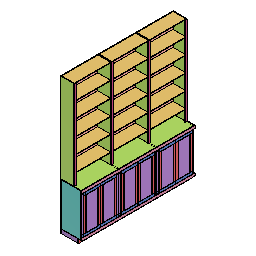
MS_BookShelves (Autodesk Fusion 360 design; units mm, degrees)
description: 68.5"x10"x0.5"
description: 10"x28"x0.5"
description: 87"x16"x0.5"
description: 29"x3"x0.5"
description: 13"x3"x0.5"
description: 6"x3"x1.5"
description: 29"x14"0.5"
description: 32.75"x13"x0.5"
description: 32.75"x29"x0.5"
description: 26.75"x3"x0.5"
description: 68.5"x29"x0.5"
description: 12.875"x2"x0.5"
description: 25.75"x2"0.5"
description: 26"x9.125"x0.25"
description: 87.5"x1.75"x0.5"
description: 16.5"x1.75"x0.5"
description: 68.5"x1.5"x0.5"
Autodesk Fusion 360 part; units mm, degrees
sketch "Sketch2" plane through (0, 0, 0) normal (0, 0, 1) x (1, 0, 0)
  line L0 (0, 0) -> (254, 0)
  line L1 (254, 0) -> (254, 2263.775)
  line L2 (254, 2263.775) -> (0, 2263.775)
  line L3 (0, 2263.775) -> (0, 0)
  line L4 (0, 0) -> (406.4, 0)
  line L5 (406.4, 0) -> (406.4, 2263.775)
  line L6 (406.4, 2263.775) -> (0, 2263.775)
  line L7 (0, 2263.775) -> (0, 0)
  line L8 (406.4, 0) -> (1338.2625, 0)
  line L9 (1338.2625, 0) -> (1338.2625, 406.4)
  line L10 (1338.2625, 406.4) -> (406.4, 406.4)
  line L11 (406.4, 406.4) -> (406.4, 0)
  dimension "d42" = 254
  dimension "d43" = 2263.775
  dimension "d45" = 406.4
  dimension "d46" = 2263.775
  dimension "d48" = 931.8625
  dimension "d49" = 406.4
  constraint horizontal L0
  constraint vertical L1
  constraint horizontal L2
  constraint vertical L3
  constraint coincident L0.start L3.end
  constraint horizontal L4
  constraint vertical L5
  constraint horizontal L6
  constraint vertical L7
  constraint horizontal L8
  constraint vertical L9
  constraint horizontal L10
  constraint vertical L11
  measures "d42" distance of L0.start L0.end
  measures "d43" distance of L0.start L2.end
  measures "d45" distance of L0.start L4.end
  measures "d46" distance of L0.start L2.end
  measures "d48" distance of L4.end L8.end
  measures "d49" distance of L4.end L10.end
sketch "Sketch1" plane through (0, 0, 0) normal (0, 0, 1) x (1, 0, 0) in component "Room"
  line L0 (0, 0) -> (3648.075, 0)
  line L1 (2259.0125, 0) -> (1363.6625, 0) construction
  line L2 (1363.6625, 0) -> (1363.6625, 46.449) construction
  line L3 (1363.6625, 46.449) -> (2259.0125, 46.449) construction
  line L4 (2259.0125, 46.449) -> (2259.0125, 0) construction
  line L5 (0, 0) -> (0, 3178.175)
  line L6 (0, 3178.175) -> (922.3375, 3178.175)
  line L7 (922.3375, 3178.175) -> (2225.675, 3178.175)
  line L8 (2225.675, 3178.175) -> (3114.675, 3178.175)
  line L9 (3114.675, 3178.175) -> (3630.6125, 3178.175)
  line L10 (0, 2403.475) -> (58.5758, 2403.475) construction
  line L11 (58.5758, 2403.475) -> (58.5758, 2317.75) construction
  line L12 (58.5758, 2317.75) -> (0, 2317.75) construction
  line L13 (0, 2317.75) -> (0, 2403.475) construction
  line L14 (140.5097, 3178.175) -> (140.5097, 2420.9375) construction
  point P0 (1363.6625, 0)
  point P1 (2259.0125, 0)
  point P2 (0, 2403.475)
  point P3 (0, 2317.75)
  dimension "d18" = 3648.075
  dimension "d19" = 895.35
  dimension "d20" = 1363.6625
  dimension "d21" = 1389.0625
  dimension "d22" = 3178.175
  dimension "d23" = 922.3375
  dimension "d24" = 1303.3375
  dimension "d25" = 889
  dimension "d26" = 515.9375
  dimension "d27" = 3630.6125
  dimension "d34" = 774.7
  dimension "d35" = 85.725
  dimension "d36" = 757.2375
  dimension "d37" = 90
  constraint coincident L0.start L5.start
  constraint horizontal L0
  constraint coincident L0 P0
  constraint coincident L0 P1
  constraint horizontal L1
  constraint vertical L2
  constraint horizontal L3
  constraint vertical L4
  constraint coincident P1 L1.start
  constraint perpendicular L0 L5
  constraint perpendicular L5 L6
  constraint parallel L6 L7
  constraint parallel L7 L8
  constraint parallel L8 L9
  constraint coincident L5 P2
  constraint coincident L5 P3
  constraint horizontal L10
  constraint vertical L11
  constraint horizontal L12
  constraint vertical L13
  constraint coincident P2 L10.start
  constraint coincident L6 L14.start
  constraint perpendicular L6 L14
  measures "d18" distance of L0.start L0.end
  measures "d19" distance of P0 P1
  measures "d20" distance of L0.start L1.end
  measures "d21" distance of L0.end P1
  measures "d22" distance of L0.start L5.end
  measures "d23" distance of L5.end L6.end
  measures "d24" distance of L6.end L7.end
  measures "d25" distance of L7.end L8.end
  measures "d26" distance of L8.end L9.end
  measures "d27" distance of L5.end L9.end
  measures "d34" distance of L5.end P2
  measures "d35" distance of P2 P3
  measures "d36" distance of L14.start L14.end
  measures "d37" angle of L6 L14
sketch "Sketch1 (2)" plane through (0, 0, 0) normal (1, 0, 0) x (0, 1, 0) in component "Shelves"
  line L0 (12.7, 2667) -> (723.9, 2667)
  line L1 (723.9, 2667) -> (723.9, 2654.3)
  line L2 (723.9, 2654.3) -> (12.7, 2654.3)
  line L3 (12.7, 2654.3) -> (12.7, 2667)
  point P0 (0, 914.4)
  point P1 (0, 927.1)
  point P2 (0, 76.2)
  point P3 (0, 2667)
  point P4 (12.7, 2667)
  dimension "d51" = 12.7
  dimension "d54" = 76.2
  dimension "d55" = 838.2
  dimension "d56" = 1739.9
  dimension "d76" = 12.7
  dimension "d77" = 711.2
  dimension "d78" = 12.7
  constraint horizontal L0
  constraint vertical L1
  constraint horizontal L2
  constraint vertical L3
  constraint coincident P4 L0.start
  measures "d51" distance of P0 P1
  measures "d54" distance of P2 origin
  measures "d55" distance of P0 P2
  measures "d56" distance of P1 P3
  measures "d76" distance of P3 P4
  measures "d77" distance of P4 L0.end
  measures "d78" distance of P4 L2.end
ref_plane "WorkPlane1" through (0, 0, 2743.2) normal (0, 0, 1) x (1, 0, 0) in component "Room"
sketch "Sketch1 (1)" plane through (0, 0, 2743.2) normal (0, 0, 1) x (1, 0, 0) in component "Room"
  line L0 (0, 0) -> (3648.075, 0) construction
  line L1 (3648.075, 0) -> (3648.075, 3178.175) construction
  line L2 (3648.075, 3178.175) -> (0, 3178.175) construction
  line L3 (0, 3178.175) -> (0, 0) construction
  dimension "d58" = 3648.075
  dimension "d59" = 3178.175
  constraint horizontal L0
  constraint vertical L1
  constraint horizontal L2
  constraint vertical L3
  constraint coincident L0.start L3.end
  measures "d58" distance of L0.start L0.end
  measures "d59" distance of L0.start L2.end
sketch "Sketch1 (3)" plane through (0, 0, 0) normal (0, 1, 0) x (1, 0, 0) in component "Shelf Sides"
  line L0 (0, -927.1) -> (260.35, -927.1)
  line L1 (260.35, -927.1) -> (260.35, -2667)
  line L2 (260.35, -2667) -> (0, -2667)
  line L3 (0, -2667) -> (0, -927.1)
  point P0 (0, -927.1)
  dimension "d60" = 260.35
  dimension "d61" = 1739.9
  constraint horizontal L0
  constraint vertical L1
  constraint horizontal L2
  constraint vertical L3
  constraint coincident P0 L0.start
  measures "d60" distance of P0 L0.end
  measures "d61" distance of P0 L2.end
extrude "Extrude1" add sketch "Sketch1 (3)" along normal blind 12.7 makes body 1 in component "Shelf Sides"
pattern_linear "00000000-0000-0000-0000-000000000000" [suppressed] in component "Shelves"
extrude "Extrude1'" add sketch "Sketch1 (2)" along normal blind 254 separate body makes body 2 in component "Shelves (1)"
sketch "Sketch1 (4)" plane through (6.35, 0, 0) normal (-1, 0, 0) x (0, -1, 0) in component "Shelf Back"
  line L0 (0, 927.1) -> (0, 2667)
  line L1 (0, 2667) -> (-12.7, 2667)
  line L2 (-12.7, 2667) -> (-12.7, 927.1)
  line L3 (-12.7, 927.1) -> (0, 927.1)
  line L4 (0, 927.1) -> (-736.6, 927.1)
  line L5 (-736.6, 927.1) -> (-736.6, 2667)
  line L6 (-736.6, 2667) -> (0, 2667)
  line L7 (0, 2667) -> (0, 927.1)
  line L8 (-723.9, 939.8) -> (-723.9, 2654.3)
  line L9 (-723.9, 2654.3) -> (-12.7, 2654.3)
  line L10 (-12.7, 2654.3) -> (-12.7, 939.8)
  line L11 (-12.7, 939.8) -> (-723.9, 939.8)
  line L12 (-723.9, 939.8) -> (-723.9, 927.1)
  line L13 (-12.7, 939.8) -> (-12.7, 927.1)
  line L14 (-723.9, 927.1) -> (-723.9, 2667)
  line L15 (-723.9, 2667) -> (-736.6, 2667)
  line L16 (-736.6, 2667) -> (-736.6, 927.1)
  line L17 (-736.6, 927.1) -> (-723.9, 927.1)
  line L18 (-723.9, 2654.3) -> (-12.7, 2654.3)
  line L19 (-12.7, 2654.3) -> (-12.7, 2667)
  line L20 (-12.7, 2667) -> (-723.9, 2667)
  line L21 (-723.9, 2667) -> (-723.9, 2654.3)
  line L22 (-723.9, 2654.3) -> (-12.7, 2654.3)
  line L23 (-12.7, 2654.3) -> (-12.7, 2667)
  line L24 (-12.7, 2667) -> (-723.9, 2667)
  line L25 (-723.9, 2667) -> (-723.9, 2654.3)
  dimension "d215" = 736.6
  dimension "d216" = 1739.9
  dimension "d217" = 12.7
  dimension "d220" = 12.7
  dimension "d221" = 12.7
  constraint horizontal L4
  constraint vertical L5
  constraint horizontal L6
  constraint vertical L7
  constraint coincident L0.start L3.end
  constraint perpendicular L11 L12
  constraint perpendicular L11 L13
  measures "d215" distance of L0.start L4.end
  measures "d216" distance of L0.start L0.end
  measures "d220" distance of L8.start L12.end
  measures "d221" distance of L10.end L2.end
extrude "Extrude1''" add sketch "Sketch1 (4)" against normal blind 6.35 separate body contours L2 L4 L11 L12 L13 L14 | L2 L8 L9 L10 L11 L14 L18 L22 makes body 3 in component "Shelf Back"
extrude "Extrude3" add sketch "Sketch1 (4)" along normal blind 6.35 separate body makes body 4 in component "Shelf Back"
pattern_linear "00000000-0000-0000-0000-000000000000'" [suppressed] in component "Shelves"
pattern_linear "00000000-0000-0000-0000-000000000000''" [suppressed] in component "Shelves"
pattern_linear "00000000-0000-0000-0000-000000000000'''" [suppressed] in component "Shelves"
pattern_linear "00000000-0000-0000-0000-000000000000''''" [suppressed] in component "Shelves"
sketch "Sketch1 (5)" plane through (0, 0, 0) normal (1, 0, 0) x (0, 1, 0) in component "Cabinet Tbl Top"
  line L0 (0, 914.4) -> (2209.8, 914.4)
  line L1 (2209.8, 914.4) -> (2209.8, 927.1)
  line L2 (2209.8, 927.1) -> (0, 927.1)
  line L3 (0, 927.1) -> (0, 914.4)
  point P0 (0, 76.2)
  point P1 (0, 914.4)
  point P2 (0, 76.2)
  dimension "d101" = 76.2
  dimension "d102" = 838.2
  dimension "d103" = 2209.8
  dimension "d104" = 12.7
  constraint vertical P0 L0.start
  constraint horizontal L0
  constraint vertical L1
  constraint horizontal L2
  constraint vertical L3
  constraint coincident P1 L0.start
  measures "d101" distance of P2 origin
  measures "d102" distance of P1 P0
  measures "d103" distance of P1 L0.end
  measures "d104" distance of P1 L2.end
extrude "Extrude1'''" add sketch "Sketch1 (5)" along normal blind 406.4 separate body makes body 5 in component "Cabinet Tbl Top"
sketch "Sketch1 (6)" plane through (0, 0, 0) normal (0, 0, 1) x (1, 0, 0) in component "Toe Guard"
  line L0 (0, 0) -> (12.7, 0)
  line L1 (12.7, 0) -> (12.7, 736.6)
  line L2 (12.7, 736.6) -> (0, 736.6)
  line L3 (0, 736.6) -> (0, 0)
  line L4 (0, 0) -> (406.4, 0)
  line L5 (342.9, 0) -> (355.6, 0)
  line L6 (355.6, 0) -> (355.6, 736.6)
  line L7 (355.6, 736.6) -> (342.9, 736.6)
  line L8 (342.9, 736.6) -> (342.9, 0)
  line L9 (12.7, 736.6) -> (342.9, 736.6)
  line L10 (342.9, 736.6) -> (342.9, 723.9)
  line L11 (342.9, 723.9) -> (12.7, 723.9)
  line L12 (12.7, 723.9) -> (12.7, 736.6)
  line L13 (12.7, 0) -> (342.9, 0)
  line L14 (342.9, 0) -> (342.9, 12.7)
  line L15 (342.9, 12.7) -> (12.7, 12.7)
  line L16 (12.7, 12.7) -> (12.7, 0)
  line L17 (120.4631, 12.7) -> (12.7, 120.4631)
  line L18 (75.5618, 3.7197) -> (3.7197, 75.5618)
  line L19 (177.8, 368.3, 0) -> (177.8, 368.3, 108.5578) construction
  point P0 (342.9, 0)
  point P1 (12.7, 12.7)
  point P2 (120.4631, 12.7)
  point P3 (12.7, 120.4631)
  point P4 (342.9, 368.3)
  point P5 (177.8, 12.7)
  point P6 (177.8, 368.3)
  dimension "d107" = 12.7
  dimension "d108" = 736.6
  dimension "d114" = 330.2
  dimension "d115" = 12.7
  dimension "d116" = 736.6
  dimension "d117" = 330.2
  dimension "d118" = 12.7
  dimension "d119" = 330.2
  dimension "d120" = 12.7
  dimension "d138" = 45
  dimension "d139" = 152.4
  constraint horizontal L0
  constraint vertical L1
  constraint horizontal L2
  constraint vertical L3
  constraint coincident L0.start L3.end
  constraint coincident P0 L4
  constraint horizontal L5
  constraint vertical L6
  constraint horizontal L7
  constraint vertical L8
  constraint coincident P0 L5.start
  constraint horizontal L9
  constraint vertical L10
  constraint horizontal L11
  constraint vertical L12
  constraint horizontal L13
  constraint vertical L14
  constraint horizontal L15
  constraint vertical L16
  constraint coincident P1 L15.end
  constraint coincident L15 P2
  constraint coincident L1 P3
  constraint coincident P2 L17.start
  constraint coincident P3 L17.end
  constraint midpoint L8 P4
  constraint midpoint L15 P5
  constraint vertical P5 P6
  measures "d107" distance of L0.start L0.end
  measures "d108" distance of L0.start L2.end
  measures "d114" distance of L0.end P0
  measures "d115" distance of P0 L5.end
  measures "d116" distance of P0 L7.end
  measures "d117" distance of L1.end L7.end
  measures "d118" distance of L1.end L11.end
  measures "d119" distance of L0.end P0
  measures "d120" distance of L0.end P1
  measures "d138" angle of L15 L17
  measures "d139" distance of P2 P3
extrude "Extrude1''''" add sketch "Sketch1 (6)" along normal blind 76.2 separate body contours L0 L1 L2 L3 L4 L12 L16 makes body 6 in component "TG F/B"
pattern_linear "00000000-0000-0000-0000-000000000000'''''" [suppressed] in component "Toe Guard"
extrude "Extrude1'''''" add sketch "Sketch1 (6)" along normal blind 76.2 separate body contours L1 L4 L8 L13 L14 L15 L16 makes body 7 in component "TG L/R"
pattern_linear "00000000-0000-0000-0000-000000000000''''''" [suppressed] in component "Toe Guard"
extrude "Extrude1''''''" add sketch "Sketch1 (6)" along normal blind 76.2 separate body contours L1 L15 L17 L18 makes body 8 in component "Toe Bracket"
component_pattern "component pattern" in component "Toe Guard"
pattern_linear "00000000-0000-0000-0000-000000000000'''''''" [suppressed] in component "W_Cabinet"
sketch "Sketch1 (7)" plane through (0, 0, 76.2) normal (0, 0, 1) x (-1, 0, 0) in component "W Cabinet Btm"
  line L0 (-12.7, 0) -> (-12.7, -736.6)
  line L1 (-12.7, -736.6) -> (0, -736.6)
  line L2 (0, -736.6) -> (0, 0)
  line L3 (0, 0) -> (-12.7, 0)
  line L4 (0, 0) -> (-406.4, 0)
  line L5 (-406.4, 0) -> (-406.4, -736.6)
  line L6 (-406.4, -736.6) -> (0, -736.6)
  line L7 (0, -736.6) -> (0, 0)
  line L8 (-393.7, -723.9) -> (-12.7, -723.9)
  line L9 (-12.7, -723.9) -> (-12.7, -12.7)
  line L10 (-12.7, -12.7) -> (-393.7, -12.7)
  line L11 (-393.7, -12.7) -> (-393.7, -723.9)
  dimension "d150" = 406.4
  dimension "d151" = 736.6
  constraint horizontal L4
  constraint vertical L5
  constraint horizontal L6
  constraint vertical L7
  constraint coincident L2.end L3.start
  measures "d150" distance of L2.end L4.end
  measures "d151" distance of L2.end L1.end
extrude "Extrude1'''''''" add sketch "Sketch1 (7)" along normal blind 12.7 separate body contours L0 L8 L9 L10 L11 makes body 9 in component "W Cabinet Btm"
extrude "Extrude2" add sketch "Sketch1 (7)" along normal blind 6.35 contours L0 L1 L2 L3 L4 L6 L7 L9 | L0 L4 L5 L6 L8 L10 L11 bodies 9 in component "W Cabinet Btm"
pattern_linear "00000000-0000-0000-0000-000000000000''''''''" [suppressed] in component "W_Cabinet"
sketch "Sketch1 (8)" plane through (0, 0, 82.55) normal (0, 0, 1) x (-1, 0, 0) in component "W Cabinet Sides"
  line L0 (-393.7, -723.9) -> (-393.7, -12.7)
  line L1 (-393.7, -12.7) -> (-12.7, -12.7)
  line L2 (-12.7, -12.7) -> (-12.7, -723.9)
  line L3 (-12.7, -723.9) -> (-393.7, -723.9)
  line L4 (0, -736.6) -> (0, 0)
  line L5 (0, 0) -> (-406.4, 0)
  line L6 (-406.4, 0) -> (-406.4, -736.6)
  line L7 (-406.4, -736.6) -> (0, -736.6)
  line L8 (-12.7, 0) -> (-393.7, 0)
  line L9 (-393.7, 0) -> (-393.7, -12.7)
  line L10 (-393.7, -12.7) -> (-12.7, -12.7)
  line L11 (-12.7, -12.7) -> (-12.7, 0)
  point P0 (-12.7, 0)
  dimension "d161" = 12.7
  dimension "d162" = 381
  dimension "d163" = 12.7
  constraint coincident L5 P0
  constraint horizontal L8
  constraint vertical L9
  constraint horizontal L10
  constraint vertical L11
  constraint coincident P0 L8.start
  measures "d161" distance of P0 L4.end
  measures "d162" distance of P0 L8.end
  measures "d163" distance of P0 L1.end
extrude "Extrude1''''''''" add sketch "Sketch1 (8)" along normal blind 831.85 separate body contours L1 L5 L8 L9 L10 L11 makes body 10 in component "W Cabinet Sides"
pattern_linear "00000000-0000-0000-0000-000000000000'''''''''" [suppressed] in component "W_Cabinet"
pattern_linear "00000000-0000-0000-0000-000000000000''''''''''" [suppressed] in component "W_Cabinet"
sketch "Sketch1 (9)" plane through (0, 0, 82.55) normal (0, 0, 1) x (-1, 0, 0) in component "W Cabinet Back"
  line L0 (-393.7, -723.9) -> (-393.7, -12.7)
  line L1 (-393.7, -12.7) -> (-12.7, -12.7)
  line L2 (-12.7, -12.7) -> (-12.7, -723.9)
  line L3 (-12.7, -723.9) -> (-393.7, -723.9)
  line L4 (0, -736.6) -> (0, 0)
  line L5 (0, 0) -> (-406.4, 0)
  line L6 (-406.4, 0) -> (-406.4, -736.6)
  line L7 (-406.4, -736.6) -> (0, -736.6)
  line L8 (0, 0) -> (-12.7, 0)
  line L9 (-12.7, 0) -> (-12.7, -736.6)
  line L10 (-12.7, -736.6) -> (0, -736.6)
  line L11 (0, -736.6) -> (0, 0)
  dimension "d178" = 12.7
  dimension "d179" = 736.6
  constraint horizontal L8
  constraint vertical L9
  constraint horizontal L10
  constraint vertical L11
  constraint coincident L4.end L5.start
  measures "d178" distance of L4.end L8.end
  measures "d179" distance of L4.end L4.start
extrude "Extrude1'''''''''" add sketch "Sketch1 (9)" along normal blind 831.85 separate body contours L2 L4 L5 L7 L8 L9 L10 L11 makes body 11 in component "W Cabinet Back"
pattern_linear "00000000-0000-0000-0000-000000000000'''''''''''" [suppressed] in component "W_Cabinet"
sketch "Sketch1 (10)" plane through (0, 0, 82.55) normal (0, 0, 1) x (-1, 0, 0) in component "W Cbnt F (T/B)"
  line L0 (-393.7, -723.9) -> (-393.7, -12.7)
  line L1 (-393.7, -12.7) -> (-12.7, -12.7)
  line L2 (-12.7, -12.7) -> (-12.7, -723.9)
  line L3 (-12.7, -723.9) -> (-393.7, -723.9)
  line L4 (0, -736.6) -> (0, 0)
  line L5 (0, 0) -> (-406.4, 0)
  line L6 (-406.4, 0) -> (-406.4, -736.6)
  line L7 (-406.4, -736.6) -> (0, -736.6)
  line L8 (-406.4, 0) -> (-393.7, 0)
  line L9 (-393.7, 0) -> (-393.7, -736.6)
  line L10 (-393.7, -736.6) -> (-406.4, -736.6)
  line L11 (-406.4, -736.6) -> (-406.4, 0)
  point P0 (-406.4, 0)
  dimension "d190" = 12.7
  dimension "d191" = 736.6
  constraint coincident L6 P0
  constraint horizontal L8
  constraint vertical L9
  constraint horizontal L10
  constraint vertical L11
  constraint coincident P0 L5.end
  measures "d190" distance of P0 L8.end
  measures "d191" distance of P0 L6.end
extrude "Extrude1''''''''''" add sketch "Sketch1 (10)" along normal blind 76.2 separate body contours L0 L5 L6 L7 L8 L9 L10 L11 makes body 12 in component "W Cbnt F (T/B)"
pattern_linear "00000000-0000-0000-0000-000000000000''''''''''''" [suppressed] in component "W Cabinet Front"
sketch "Sketch1 (11)" plane through (0, 0, 158.75) normal (0, 0, 1) x (-1, 0, 0) in component "W Cbnt F (L/R)"
  line L0 (-406.4, -736.6) -> (-393.7, -736.6)
  line L1 (-393.7, -736.6) -> (-393.7, 0)
  line L2 (-393.7, 0) -> (-406.4, 0)
  line L3 (-406.4, 0) -> (-406.4, -736.6)
  line L4 (-406.4, 0) -> (-393.7, 0)
  line L5 (-393.7, 0) -> (-393.7, -76.2)
  line L6 (-393.7, -76.2) -> (-406.4, -76.2)
  line L7 (-406.4, -76.2) -> (-406.4, 0)
  dimension "d199" = 12.7
  dimension "d200" = 76.2
  constraint horizontal L4
  constraint vertical L5
  constraint horizontal L6
  constraint vertical L7
  constraint coincident L2.end L3.start
  measures "d199" distance of L2.end L1.end
  measures "d200" distance of L2.end L6.end
extrude "Extrude1'''''''''''" add sketch "Sketch1 (11)" along normal blind 679.45 separate body contours L1 L2 L3 L4 L5 L6 L7 makes body 13 in component "W Cbnt F (L/R)"
pattern_linear "00000000-0000-0000-0000-000000000000'''''''''''''" [suppressed] in component "W Cabinet Front"
pattern_linear "00000000-0000-0000-0000-000000000000''''''''''''''" [suppressed] in component "W_Cabinet"
ref_plane "WorkPlane1" through (406.4, 368.3, 120.65) normal (1, 0, 0) x (0, 1, 0) in component "W Doors"
sketch "Sketch1 (12)" plane through (406.4, 0, 0) normal (1, 0, 0) x (0, 1, 0) in component "W Door"
  line L0 (0, 838.2) -> (736.6, 838.2)
  line L1 (736.6, 838.2) -> (736.6, 914.4)
  line L2 (736.6, 914.4) -> (0, 914.4)
  line L3 (0, 914.4) -> (0, 838.2)
  line L4 (44.45, 869.95) -> (95.25, 869.95)
  line L5 (95.25, 869.95) -> (95.25, 549.275)
  line L6 (95.25, 549.275) -> (44.45, 549.275)
  line L7 (44.45, 549.275) -> (44.45, 869.95)
  point P0 (44.45, 869.95)
  dimension "d233" = 44.45
  dimension "d237" = 44.45
  dimension "d238" = 50.8
  dimension "d239" = 320.675
  constraint horizontal L4
  constraint vertical L5
  constraint horizontal L6
  constraint vertical L7
  constraint coincident P0 L4.start
  measures "d233" distance of L2 P0
  measures "d237" distance of L3 P0
  measures "d238" distance of P0 L4.end
  measures "d239" distance of P0 L6.end
sketch "Sketch1 (13)" plane through (406.4, 0, 0) normal (1, 0, 0) x (0, 1, 0) in component "W_Door_TB"
  line L0 (0, 838.2) -> (736.6, 838.2)
  line L1 (736.6, 838.2) -> (736.6, 914.4)
  line L2 (736.6, 914.4) -> (0, 914.4)
  line L3 (0, 914.4) -> (0, 838.2)
  line L4 (41.275, 869.95) -> (361.95, 869.95)
  line L5 (361.95, 869.95) -> (361.95, 819.15)
  line L6 (361.95, 819.15) -> (41.275, 819.15)
  line L7 (41.275, 819.15) -> (41.275, 869.95)
  line L8 (368.3, 914.4) -> (368.3, 82.3581) construction
  point P0 (41.275, 869.95)
  dimension "d240" = 44.45
  dimension "d244" = 320.675
  dimension "d245" = 50.8
  constraint horizontal L4
  constraint vertical L5
  constraint horizontal L6
  constraint vertical L7
  constraint coincident P0 L4.start
  constraint midpoint L2 L8.start
  constraint perpendicular L0 L8
  measures "d240" distance of L2 P0
  measures "d244" distance of P0 L4.end
  measures "d245" distance of P0 L6.end
extrude "Extrude1''''''''''''" add sketch "Sketch1 (13)" along normal blind 12.7 separate body contours L0 L4 L5 L7 | L0 L5 L6 L7 makes body 14 in component "W_Door_TB"
pattern_linear "00000000-0000-0000-0000-000000000000'''''''''''''''" [suppressed] in component "W Door"
sketch "Sketch1 (14)" plane through (419.1, 0, 0) normal (1, 0, 0) x (0, 1, 0) in component "W_Door_LR"
  line L0 (41.275, 819.15) -> (361.95, 819.15)
  line L1 (361.95, 819.15) -> (361.95, 869.95)
  line L2 (361.95, 869.95) -> (41.275, 869.95)
  line L3 (41.275, 869.95) -> (41.275, 819.15)
  line L4 (41.275, 819.15) -> (92.075, 819.15)
  line L5 (92.075, 819.15) -> (92.075, 177.8)
  line L6 (92.075, 177.8) -> (41.275, 177.8)
  line L7 (41.275, 177.8) -> (41.275, 819.15)
  dimension "d258" = 50.8
  dimension "d259" = 641.35
  constraint horizontal L4
  constraint vertical L5
  constraint horizontal L6
  constraint vertical L7
  constraint coincident L0.start L3.end
  measures "d258" distance of L0.start L4.end
  measures "d259" distance of L0.start L6.end
extrude "Extrude1'''''''''''''" add sketch "Sketch1 (14)" against normal blind 12.7 separate body contours L0 L4 L5 L6 L7 makes body 15 in component "W_Door_LR"
pattern_linear "00000000-0000-0000-0000-000000000000''''''''''''''''" [suppressed] in component "W Door"
sketch "Sketch1 (15)" plane through (419.1, 0, 0) normal (1, 0, 0) x (0, 1, 0) in component "W_Door_Centr"
  line L0 (41.275, 177.8) -> (92.075, 177.8)
  line L1 (92.075, 177.8) -> (92.075, 819.15)
  line L2 (92.075, 819.15) -> (41.275, 819.15)
  line L3 (41.275, 819.15) -> (41.275, 177.8)
  line L4 (88.9, 822.325) -> (314.325, 822.325)
  line L5 (314.325, 822.325) -> (314.325, 174.625)
  line L6 (314.325, 174.625) -> (88.9, 174.625)
  line L7 (88.9, 174.625) -> (88.9, 822.325)
  point P0 (88.9, 822.325)
  dimension "d269" = 3.175
  dimension "d270" = 3.175
  dimension "d271" = 225.425
  dimension "d272" = 647.7
  constraint horizontal L4
  constraint vertical L5
  constraint horizontal L6
  constraint vertical L7
  constraint coincident P0 L4.start
  measures "d269" distance of L2 P0
  measures "d270" distance of L1 P0
  measures "d271" distance of P0 L4.end
  measures "d272" distance of P0 L6.end
extrude "Extrude1''''''''''''''" add sketch "Sketch1 (15)" against normal blind 6.35 separate body contours L0 L1 L2 L7 | L0 L1 L2 L4 L5 L6 L7 makes body 16 in component "W_Door_Centr"
pattern_linear "00000000-0000-0000-0000-000000000000'''''''''''''''''" [suppressed] in component "W Door"
pattern_linear "00000000-0000-0000-0000-000000000000''''''''''''''''''" [suppressed] in component "W Doors"
sketch "Sketch1 (16)" plane through (406.4, 0, 0) normal (1, 0, 0) x (0, 1, 0) in component "cbnt_W_trim_W"
  line L0 (0, 927.1) -> (0, 914.4)
  line L1 (0, 914.4) -> (2209.8, 914.4)
  line L2 (2209.8, 914.4) -> (2209.8, 927.1)
  line L3 (2209.8, 927.1) -> (0, 927.1)
  line L4 (0, 927.1) -> (2222.5, 927.1)
  line L5 (2222.5, 927.1) -> (2222.5, 876.3)
  line L6 (2222.5, 876.3) -> (0, 876.3)
  line L7 (0, 876.3) -> (0, 927.1)
  dimension "d283" = 2222.5
  dimension "d284" = 50.8
  constraint horizontal L4
  constraint vertical L5
  constraint horizontal L6
  constraint vertical L7
  constraint coincident L0.start L3.end
  measures "d283" distance of L0.start L4.end
  measures "d284" distance of L0.start L6.end
extrude "Extrude1'''''''''''''''" add sketch "Sketch1 (16)" along normal blind 12.7 separate body makes body 17 in component "cbnt_W_trim_W"
chamfer "Chamfer1" distance 12.7 angle 45 1 edges at (406.4, 2222.5, 901.7) on bodies 17 in component "cbnt_W_trim_W"
sketch "Sketch1 (17)" plane through (0, 2209.8, 0) normal (0, 1, 0) x (-1, 0, 0) in component "cbnt_W_trim_N"
  line L0 (0, 914.4) -> (0, 927.1)
  line L1 (0, 927.1) -> (-406.4, 927.1)
  line L2 (-406.4, 927.1) -> (-406.4, 914.4)
  line L3 (-406.4, 914.4) -> (0, 914.4)
  line L4 (0, 927.1) -> (-419.1, 927.1)
  line L5 (-419.1, 927.1) -> (-419.1, 876.3)
  line L6 (-419.1, 876.3) -> (0, 876.3)
  line L7 (0, 876.3) -> (0, 927.1)
  dimension "d290" = 419.1
  dimension "d291" = 50.8
  constraint horizontal L4
  constraint vertical L5
  constraint horizontal L6
  constraint vertical L7
  constraint coincident L0.end L1.start
  measures "d290" distance of L0.end L4.end
  measures "d291" distance of L0.end L6.end
extrude "Extrude1''''''''''''''''" add sketch "Sketch1 (17)" along normal blind 12.7 separate body makes body 18 in component "cbnt_W_trim_N"
chamfer "Chamfer1'" distance 12.7 angle 45 1 edges at (419.1, 2209.8, 901.7) on bodies 18 in component "cbnt_W_trim_N"
pattern_linear "00000000-0000-0000-0000-000000000000'''''''''''''''''''" [suppressed] in component "W_Cabinet"
sketch "Sketch1 (18)" plane through (260.35, 0, 0) normal (1, 0, 0) x (0, 1, 0) in component "Molding"
  line L0 (0, 2667) -> (0, 927.1)
  line L1 (0, 927.1) -> (12.7, 927.1)
  line L2 (12.7, 927.1) -> (12.7, 2667)
  line L3 (12.7, 2667) -> (0, 2667)
  line L4 (0, 2666.9746) -> (38.1, 2666.9746)
  line L5 (38.1, 2666.9746) -> (38.1, 927.0746)
  line L6 (38.1, 927.0746) -> (0, 927.0746)
  line L7 (0, 927.0746) -> (0, 2666.9746)
  line L8 (2171.7, 2666.9746) -> (2209.8, 2666.9746)
  line L9 (2209.8, 2666.9746) -> (2209.8, 927.0746)
  line L10 (2209.8, 927.0746) -> (2171.7, 927.0746)
  line L11 (2171.7, 927.0746) -> (2171.7, 2666.9746)
  point P0 (0, 2666.9746)
  point P1 (2171.7, 2666.9746)
  dimension "d302" = 0.0254
  dimension "d303" = 38.1
  dimension "d304" = 1739.9
  dimension "d305" = 38.1
  dimension "d306" = 1739.9
  dimension "d307" = 2209.8
  constraint coincident L0 P0
  constraint horizontal L4
  constraint vertical L5
  constraint horizontal L6
  constraint vertical L7
  constraint coincident P0 L4.start
  constraint horizontal L8
  constraint vertical L9
  constraint horizontal L10
  constraint vertical L11
  constraint coincident P1 L8.start
  constraint collinear L4 L8
  measures "d302" distance of L0.start P0
  measures "d303" distance of P0 L4.end
  measures "d304" distance of P0 L6.end
  measures "d305" distance of P1 L8.end
  measures "d306" distance of P1 L10.end
  measures "d307" distance of P0 L8.end
extrude "Extrude1'''''''''''''''''" add sketch "Sketch1 (18)" along normal blind 12.7 separate body contours L0 L1 L2 L4 L7 | L1 L2 L4 L5 L6 L7 makes body 19 in component "Shlf_Molding"
pattern_linear "00000000-0000-0000-0000-000000000000''''''''''''''''''''" [suppressed] in component "Molding"
sketch "Sketch3" plane through (406.4, 0, 0) normal (1, 0, 0) x (0, 1, 0) in component "cbnt_W_trim_W_TB"
  line L0 (0, 838.2) -> (736.6, 838.2)
  line L1 (736.6, 838.2) -> (736.6, 914.4)
  line L2 (736.6, 914.4) -> (0, 914.4)
  line L3 (0, 914.4) -> (0, 838.2)
  line L4 (0, 876.3) -> (38.1, 876.3)
  line L5 (38.1, 876.3) -> (38.1, 120.65)
  line L6 (38.1, 120.65) -> (0, 120.65)
  line L7 (0, 120.65) -> (0, 876.3)
  point P0 (0, 876.3)
  dimension "d316" = 38.1
  dimension "d319" = 755.65
  dimension "d320" = 38.1
  constraint coincident L3 P0
  constraint horizontal L4
  constraint vertical L5
  constraint horizontal L6
  constraint vertical L7
  constraint coincident P0 L4.start
  measures "d316" distance of L2.end P0
  measures "d319" distance of P0 L6.end
  measures "d320" distance of L5 L7
sketch "Sketch4" plane through (0, 0, 0) normal (1, 0, 0) x (0, 1, 0)
  line L0 (-2337.1561, -250.9121) -> (-241.5061, -257.4352) construction
  line L1 (-241.5061, -257.4352) -> (-234.1991, 2090.0497) construction
  line L2 (-234.1991, 2090.0497) -> (-2329.8491, 2096.5728) construction
  line L3 (-2329.8491, 2096.5728) -> (-2337.1561, -250.9121) construction
  dimension "d321" = 50.8
component "Shelves" placed x (1, 0, 0) y (0, 1, 0) z (0, 0, 1) at (0, 0, 0)
component "Room" placed x (1, 0, 0) y (0, 1, 0) z (0, 0, 1) at (0, 0, 0)
component "W_Cabinet" placed x (1, 0, 0) y (0, 1, 0) z (0, 0, 1) at (0, 0, 0)
component "Shelf Sides" placed x (1, 0, 0) y (0, 1, 0) z (0, 0, 1) at (0, 0, 0) in component "Shelves"
component "Shelf Sides" placed x (1, 0, 0) y (0, 1, 0) z (0, 0, 1) at (0, 723.9, 0) in component "Shelves"
component "Shelves (1)" placed x (1, 0, 0) y (0, 1, 0) z (0, 0, 1) at (6.35, 0, 0) in component "Shelves"
component "Shelf Back" placed x (1, 0, 0) y (0, 1, 0) z (0, 0, 1) at (0, 0, 0) in component "Shelves"
component "Shelf Back" placed x (1, 0, 0) y (0, 1, 0) z (0, 0, 1) at (0, 736.6, 0) in component "Shelves"
component "Shelf Back" placed x (1, 0, 0) y (0, 1, 0) z (0, 0, 1) at (0, 1473.2, 0) in component "Shelves"
component "Shelf Sides" placed x (1, 0, 0) y (0, 1, 0) z (0, 0, 1) at (0, 736.6, 0) in component "Shelves"
component "Shelf Sides" placed x (1, 0, 0) y (0, 1, 0) z (0, 0, 1) at (0, 1460.5, 0) in component "Shelves"
component "Shelf Sides" placed x (1, 0, 0) y (0, 1, 0) z (0, 0, 1) at (0, 1473.2, 0) in component "Shelves"
component "Shelf Sides" placed x (1, 0, 0) y (0, 1, 0) z (0, 0, 1) at (0, 2197.1, 0) in component "Shelves"
component "Shelves (1)" placed x (1, 0, 0) y (0, 1, 0) z (0, 0, 1) at (6.35, 736.6, 0) in component "Shelves"
component "Shelves (1)" placed x (1, 0, 0) y (0, 1, 0) z (0, 0, 1) at (6.35, 1473.2, 0) in component "Shelves"
component "Shelves (1)" placed x (1, 0, 0) y (0, 1, 0) z (0, 0, 1) at (6.35, 0, -304.8) in component "Shelves"
component "Shelves (1)" placed x (1, 0, 0) y (0, 1, 0) z (0, 0, 1) at (6.35, 736.6, -304.8) in component "Shelves"
component "Shelves (1)" placed x (1, 0, 0) y (0, 1, 0) z (0, 0, 1) at (6.35, 1473.2, -304.8) in component "Shelves"
component "Shelves (1)" placed x (1, 0, 0) y (0, 1, 0) z (0, 0, 1) at (6.35, 0, -609.6) in component "Shelves"
component "Shelves (1)" placed x (1, 0, 0) y (0, 1, 0) z (0, 0, 1) at (6.35, 736.6, -609.6) in component "Shelves"
component "Shelves (1)" placed x (1, 0, 0) y (0, 1, 0) z (0, 0, 1) at (6.35, 1473.2, -609.6) in component "Shelves"
component "Shelves (1)" placed x (1, 0, 0) y (0, 1, 0) z (0, 0, 1) at (6.35, 0, -914.4) in component "Shelves"
component "Shelves (1)" placed x (1, 0, 0) y (0, 1, 0) z (0, 0, 1) at (6.35, 736.6, -914.4) in component "Shelves"
component "Shelves (1)" placed x (1, 0, 0) y (0, 1, 0) z (0, 0, 1) at (6.35, 1473.2, -914.4) in component "Shelves"
component "Shelves (1)" placed x (1, 0, 0) y (0, 1, 0) z (0, 0, 1) at (6.35, 0, -1219.2) in component "Shelves"
component "Shelves (1)" placed x (1, 0, 0) y (0, 1, 0) z (0, 0, 1) at (6.35, 736.6, -1219.2) in component "Shelves"
component "Shelves (1)" placed x (1, 0, 0) y (0, 1, 0) z (0, 0, 1) at (6.35, 1473.2, -1219.2) in component "Shelves"
component "Shelves (1)" placed x (1, 0, 0) y (0, 1, 0) z (0, 0, 1) at (6.35, 0, -1524) in component "Shelves"
component "Shelves (1)" placed x (1, 0, 0) y (0, 1, 0) z (0, 0, 1) at (6.35, 736.6, -1524) in component "Shelves"
component "Shelves (1)" placed x (1, 0, 0) y (0, 1, 0) z (0, 0, 1) at (6.35, 1473.2, -1524) in component "Shelves"
component "Molding" placed x (1, 0, 0) y (0, 1, 0) z (0, 0, 1) at (0, 0, 0) in component "Shelves"
component "Cabinet Tbl Top" placed x (1, 0, 0) y (0, 1, 0) z (0, 0, 1) at (0, 0, 0) in component "W_Cabinet"
component "Toe Guard" placed x (1, 0, 0) y (0, 1, 0) z (0, 0, 1) at (0, 0, 0) in component "W_Cabinet"
component "Toe Guard" placed x (1, 0, 0) y (0, 1, 0) z (0, 0, 1) at (0, 736.6, 0) in component "W_Cabinet"
component "Toe Guard" placed x (1, 0, 0) y (0, 1, 0) z (0, 0, 1) at (0, 1473.2, 0) in component "W_Cabinet"
component "W Cabinet Btm" placed x (1, 0, 0) y (0, 1, 0) z (0, 0, 1) at (0, 0, 0) in component "W_Cabinet"
component "W Cabinet Btm" placed x (1, 0, 0) y (0, 1, 0) z (0, 0, 1) at (0, 736.6, 0) in component "W_Cabinet"
component "W Cabinet Btm" placed x (1, 0, 0) y (0, 1, 0) z (0, 0, 1) at (0, 1473.2, 0) in component "W_Cabinet"
component "W Cabinet Sides" placed x (1, 0, 0) y (0, 1, 0) z (0, 0, 1) at (0, 0, 0) in component "W_Cabinet"
component "W Cabinet Sides" placed x (1, 0, 0) y (0, 1, 0) z (0, 0, 1) at (0, 723.9, 0) in component "W_Cabinet"
component "W Cabinet Sides" placed x (1, 0, 0) y (0, 1, 0) z (0, 0, 1) at (0, 736.6, 0) in component "W_Cabinet"
component "W Cabinet Sides" placed x (1, 0, 0) y (0, 1, 0) z (0, 0, 1) at (0, 1460.5, 0) in component "W_Cabinet"
component "W Cabinet Sides" placed x (1, 0, 0) y (0, 1, 0) z (0, 0, 1) at (0, 1473.2, 0) in component "W_Cabinet"
component "W Cabinet Sides" placed x (1, 0, 0) y (0, 1, 0) z (0, 0, 1) at (0, 2197.1, 0) in component "W_Cabinet"
component "W Cabinet Back" placed x (1, 0, 0) y (0, 1, 0) z (0, 0, 1) at (0, 0, 0) in component "W_Cabinet"
component "W Cabinet Back" placed x (1, 0, 0) y (0, 1, 0) z (0, 0, 1) at (0, 736.6, 0) in component "W_Cabinet"
component "W Cabinet Back" placed x (1, 0, 0) y (0, 1, 0) z (0, 0, 1) at (0, 1473.2, 0) in component "W_Cabinet"
component "W Cabinet Front" placed x (1, 0, 0) y (0, 1, 0) z (0, 0, 1) at (0, 0, 0) in component "W_Cabinet"
component "W Cabinet Front" placed x (1, 0, 0) y (0, 1, 0) z (0, 0, 1) at (0, 736.6, 0) in component "W_Cabinet"
component "W Cabinet Front" placed x (1, 0, 0) y (0, 1, 0) z (0, 0, 1) at (0, 1473.2, 0) in component "W_Cabinet"
component "W Doors" placed x (1, 0, 0) y (0, 1, 0) z (0, 0, 1) at (0, 0, 0) in component "W_Cabinet"
component "cbnt_W_trim_W" placed x (1, 0, 0) y (0, 1, 0) z (0, 0, 1) at (0, 0, 0) in component "W_Cabinet"
component "cbnt_W_trim_N" placed x (1, 0, 0) y (0, 1, 0) z (0, 0, 1) at (0, 0, 0) in component "W_Cabinet"
component "cbnt_W_trim_W" placed x (1, 0, 0) y (0, 1, 0) z (0, 0, 1) at (0, 0, -806.45) in component "W_Cabinet"
component "cbnt_W_trim_N" placed x (1, 0, 0) y (0, 1, 0) z (0, 0, 1) at (0, 0, -806.45) in component "W_Cabinet"
component "cbnt_W_trim_W_TB" placed x (1, 0, 0) y (0, 1, 0) z (0, 0, 1) at (0, 0, 0) in component "W_Cabinet"
component "TG F/B" placed x (1, 0, 0) y (0, 1, 0) z (0, 0, 1) at (0, 0, 0) in component "Toe Guard"
component "TG F/B" placed x (1, 0, 0) y (0, 1, 0) z (0, 0, 1) at (342.9, 0, 0) in component "Toe Guard"
component "TG L/R" placed x (1, 0, 0) y (0, 1, 0) z (0, 0, 1) at (0, 0, 0) in component "Toe Guard"
component "TG L/R" placed x (1, 0, 0) y (0, 1, 0) z (0, 0, 1) at (0, 723.9, 0) in component "Toe Guard"
component "Toe Bracket" placed x (1, 0, 0) y (0, 1, 0) z (0, 0, 1) at (0, 0, 0) in component "Toe Guard"
component "Toe Bracket" placed x (0, 1, 0) y (-1, 0, 0) z (0, 0, 1) at (355.6, 0, 0) in component "Toe Guard"
component "Toe Bracket" placed x (-1, 0, 0) y (0, -1, 0) z (0, 0, 1) at (355.6, 736.6, 0) in component "Toe Guard"
component "Toe Bracket" placed x (0, -1, 0) y (1, 0, 0) z (0, 0, 1) at (0, 736.6, 0) in component "Toe Guard"
component "W Cbnt F (T/B)" placed x (1, 0, 0) y (0, 1, 0) z (0, 0, 1) at (0, 0, 0) in component "W Cabinet Front"
component "W Cbnt F (T/B)" placed x (1, 0, 0) y (0, 1, 0) z (0, 0, 1) at (0, 0, 755.65) in component "W Cabinet Front"
component "W Cbnt F (L/R)" placed x (1, 0, 0) y (0, 1, 0) z (0, 0, 1) at (0, 0, 0) in component "W Cabinet Front"
component "W Cbnt F (L/R)" placed x (1, 0, 0) y (0, 1, 0) z (0, 0, 1) at (0, 660.4, 0) in component "W Cabinet Front"
component "W Door" placed x (1, 0, 0) y (0, 1, 0) z (0, 0, 1) at (0, 0, 0) in component "W Doors"
component "W Door" placed x (1, 0, 0) y (0, 1, 0) z (0, 0, 1) at (0, 736.6, 0) in component "W Doors"
component "W Door" placed x (1, 0, 0) y (0, 1, 0) z (0, 0, 1) at (0, 1473.2, 0) in component "W Doors"
component "W_Door_TB" placed x (1, 0, 0) y (0, 1, 0) z (0, 0, 1) at (0, 0, 0) in component "W Door"
component "W_Door_TB" placed x (1, 0, 0) y (0, 1, 0) z (0, 0, 1) at (0, 0, -692.15) in component "W Door"
component "W_Door_LR" placed x (1, 0, 0) y (0, 1, 0) z (0, 0, 1) at (0, 0, 0) in component "W Door"
component "W_Door_LR" placed x (1, 0, 0) y (0, 1, 0) z (0, 0, 1) at (0, 269.875, 0) in component "W Door"
component "W_Door_Centr" placed x (1, 0, 0) y (0, 1, 0) z (0, 0, 1) at (6.35, 0, 0) in component "W Door"
component "W_Door_TB" placed x (1, 0, 0) y (0, 1, 0) z (0, 0, 1) at (0, 327.025, 0) in component "W Door"
component "W_Door_TB" placed x (1, 0, 0) y (0, 1, 0) z (0, 0, 1) at (0, 327.025, -692.15) in component "W Door"
component "W_Door_LR" placed x (1, 0, 0) y (0, 1, 0) z (0, 0, 1) at (0, 327.025, 0) in component "W Door"
component "W_Door_LR" placed x (1, 0, 0) y (0, 1, 0) z (0, 0, 1) at (0, 596.9, 0) in component "W Door"
component "W_Door_Centr" placed x (1, 0, 0) y (0, 1, 0) z (0, 0, 1) at (0, 327.025, 0) in component "W Door"
component "Shlf_Molding" placed x (1, 0, 0) y (0, 1, 0) z (0, 0, 1) at (0, 0, 0) in component "Molding"
component "Shlf_Molding" placed x (1, 0, 0) y (0, 1, 0) z (0, 0, 1) at (0, 723.9, 0) in component "Molding"
component "Shlf_Molding" placed x (1, 0, 0) y (0, 1, 0) z (0, 0, 1) at (0, 1447.8, 0) in component "Molding"
component "Shlf_Molding" placed x (1, 0, 0) y (0, 1, 0) z (0, 0, 1) at (0, 2171.7, 0) in component "Molding"
equation "room_W_wall = 10'-0\" + 5\" + 0.125 in"
equation "room_distance_to_ceiling = 9 ft"
equation "room_shelves_depth = 11\" + 0'- 1/16\""
equation "room_shelves_width = 5'-0\" + 0'- 9/16\""
equation "room_shelves_height = 58.75 in"
equation "room_doors_left = 2'-0\" + 5\" + 0'- 13/16\""
equation "room_doors_right = room_doors_left"
equation "room_doorframe_left = 2'-0\" + 11\""
equation "room_doorframe_right = room_doorframe_left"
equation "room_NS_wall = 11'-0\" + 10.75 in"
equation "room_S_wall_right = 4'-0\" + 5\" + 0'- 11/16\""
equation "room_S_wall_left = 4'-0\" + 6\" + 0'- 11/16\""
equation "room_S_wall_window = 2'-0\" + 11.25 in"
equation "room_S_wall_total = room_S_wall_left + room_S_wall_right + room_S_wall_window"
equation "room_N_wall_p1 = 3'-0\" + 0'- 5/16\""
equation "room_N_wall_p2 = 4'-0\" + 3\" + 0'- 5/16\""
equation "room_N_wall_p3 = 1'-0\" + 8\" + 0'- 5/16\""
equation "d18 = room_S_wall_total"
equation "d19 = room_S_wall_window"
equation "d20 = room_S_wall_right"
equation "d22 = room_W_wall"
equation "d23 = room_N_wall_p1"
equation "d24 = room_N_wall_p2"
equation "d25 = room_doorframe_right"
equation "d26 = room_N_wall_p3"
equation "room_W_outlet_NWallToRight = 2'-0\" + 6.5 in"
equation "room_W_outlet_floorToBtm = 11\" + 0'- 5/8\""
equation "room_W_outlet_floorToTop = 1'-0\" + 4\" + 0'- 11/16\""
equation "room_W_outlet_NWallToLeft = 2'-0\" + 9\" + 0'- 7/8\""
equation "room_W_outlet_length = room_W_outlet_floorToTop - room_W_outlet_floorToBtm"
equation "room_W_outlet_width = room_W_outlet_NWallToLeft - room_W_outlet_NWallToRight"
equation "d34 = room_W_outlet_NWallToRight"
equation "d35 = room_W_outlet_width"
equation "d36 = room_doors_left"
equation "material_thickness = 0.5 in"
equation "shlf_depth = 10 in"
equation "cabinet_height = 3'-0\" - cabinet_toe_guard"
equation "shlf_W_ttl_width = room_W_wall - 36\""
equation "d42 = shlf_depth"
equation "d43 = shlf_W_ttl_width"
equation "cabinet_depth = shlf_depth + 6\""
equation "d45 = cabinet_depth"
equation "d46 = shlf_W_ttl_width"
equation "shlf_S_ttl_width = room_S_wall_right - cabinet_depth - 1 in"
equation "d48 = shlf_S_ttl_width"
equation "d49 = cabinet_depth"
equation "d51 = material_thickness"
equation "shlf_ttl_height = room_distance_to_ceiling - cabinet_height - material_thickness - cabinet_toe_guard - 3\""
equation "cabinet_toe_guard = material_toe_width"
equation "d54 = cabinet_toe_guard"
equation "d55 = cabinet_height"
equation "d56 = shlf_ttl_height"
equation "d57 = room_distance_to_ceiling"
equation "d58 = room_S_wall_total"
equation "d59 = room_W_wall"
equation "d60 = shlf_W_sides_width"
equation "d61 = shlf_W_side_length"
equation "d62 = material_thickness"
equation "shlf_W_NumOfSections = 3"
equation "shlf_W_numOfSides = shlf_W_NumOfSections * 2"
equation "shlf_W_ttl_SidesThickness = shlf_W_numOfSides * material_thickness"
equation "shlf_W_shelf_length = floor(( shlf_W_ttl_width - shlf_W_ttl_SidesThickness ) / shlf_W_NumOfSections)"
equation "shlf_W_distanceBTWShelves = 12 in"
equation "shlf_W_numOfShelves = floor(shlf_ttl_height / shlf_W_distanceBTWShelves) + 1"
equation "d76 = material_thickness"
equation "d77 = shlf_W_shelf_length"
equation "d78 = material_thickness"
equation "d79 = shlf_depth"
equation "d82 = shlf_W_NumOfSections"
equation "d84 = shlf_W_shelf_length + ( material_thickness * 2 )"
equation "d85 = shlf_W_numOfShelves"
equation "d87 = -shlf_W_distanceBTWShelves"
equation "d96 = shlf_W_shelf_length + material_thickness"
equation "d98 = shlf_W_NumOfSections"
equation "d100 = shlf_W_shelf_length + ( material_thickness * 2 )"
equation "d101 = cabinet_toe_guard"
equation "d102 = cabinet_height"
equation "d103 = cabinet_W_tblTopLength"
equation "d104 = material_thickness"
equation "d105 = cabinet_depth"
equation "d107 = material_thickness"
equation "d108 = toe_W_length"
equation "toe_W_length = shlf_W_shelf_length + ( material_thickness * 2 )"
equation "toe_W_width = cabinet_depth - cabinet_toe_guard"
equation "d114 = toe_W_width"
equation "d115 = material_thickness"
equation "d116 = toe_W_length"
equation "d117 = toe_W_width"
equation "d118 = material_thickness"
equation "d119 = toe_W_width"
equation "d120 = material_thickness"
equation "d121 = cabinet_toe_guard"
equation "d126 = toe_W_width + material_thickness"
equation "d127 = cabinet_toe_guard"
equation "d132 = toe_W_length - material_thickness"
equation "material_toe_width = 3.0 in"
equation "material_toe_thickness = 1.5 in"
equation "toe_bracket = 6 in"
equation "d139 = toe_bracket"
equation "d140 = -material_toe_thickness"
equation "d141 = cabinet_toe_guard"
equation "d146 = shlf_W_NumOfSections"
equation "d148 = toe_W_length"
equation "cabinet_W_tblTopLength = ( shlf_W_shelf_length + ( material_thickness * 2 ) ) * 3"
equation "d150 = cabinet_W_btm_width"
equation "d151 = cabinet_W_btm_length"
equation "d152 = -material_thickness"
equation "d153 = material_thickness"
equation "d155 = material_thickness / 2"
equation "d158 = shlf_W_NumOfSections"
equation "d160 = toe_W_length"
equation "d161 = material_thickness"
equation "d162 = cabinet_W_side_width"
equation "d163 = material_thickness"
equation "cabinet_W_side_width = cabinet_depth - ( material_thickness * 2 )"
equation "cabinet_W_side_length = cabinet_height - ( material_thickness / 2 )"
equation "d166 = cabinet_W_side_length"
equation "d171 = toe_W_length - material_thickness"
equation "d173 = shlf_W_NumOfSections"
equation "d175 = toe_W_length"
equation "cabinet_W_back_length = cabinet_height - ( material_thickness / 2 )"
equation "cabinet_W_back_width = toe_W_length"
equation "d178 = material_thickness"
equation "d179 = cabinet_W_back_width"
equation "d180 = cabinet_W_back_length"
equation "d183 = shlf_W_NumOfSections"
equation "d185 = toe_W_length"
equation "cabinet_W_btm_width = cabinet_depth"
equation "cabinet_W_btm_length = toe_W_length"
equation "cabinet_W_front_TB_length = cabinet_W_btm_length"
equation "d190 = material_thickness"
equation "d191 = cabinet_W_front_TB_length"
equation "cabinet_W_front_width = cabinet_bezzle"
equation "d193 = cabinet_W_front_width"
equation "d197 = -cabinet_height + cabinet_W_front_width + ( material_thickness / 2 )"
equation "d199 = material_thickness"
equation "d200 = cabinet_W_front_width"
equation "cabinet_W_front_LR_length = cabinet_W_side_length - ( cabinet_W_front_width * 2 )"
equation "d202 = cabinet_W_front_LR_length"
equation "cabinet_bezzle = 3 in"
equation "d207 = cabinet_W_btm_length - cabinet_W_front_width"
equation "d209 = shlf_W_NumOfSections"
equation "d211 = cabinet_W_btm_length"
equation "shlf_W_back_width = shlf_W_shelf_length + ( material_thickness * 2 )"
equation "shlf_W_back_length = shlf_ttl_height"
equation "d215 = shlf_W_back_width"
equation "d216 = shlf_W_back_length"
equation "d217 = material_thickness"
equation "d218 = -material_thickness / 2"
equation "d224 = material_thickness / 2"
equation "shlf_W_sides_width = shlf_depth + ( material_thickness / 2 )"
equation "shlf_W_side_length = shlf_ttl_height"
equation "d229 = shlf_W_NumOfSections"
equation "d231 = shlf_W_shelf_length + ( material_thickness * 2 )"
equation "d233 = cabinet_W_door_offset"
equation "cabinet_W_door_offset = ( cabinet_bezzle / 2 ) + 0.25 in"
equation "cabinet_W_door_TB_length = ( cabinet_W_front_TB_length / 2 ) - cabinet_W_door_offset - ( cabinet_W_doors_spaceBTWDoors / 2 )"
equation "cabinet_W_door_TB_width = cabinet_door_bezzle"
equation "d237 = cabinet_W_door_offset"
equation "d238 = cabinet_W_door_TB_width"
equation "d239 = cabinet_W_door_TB_length"
equation "d240 = cabinet_W_door_offset"
equation "cabinet_W_doors_spaceBTWDoors = 0.25 in"
equation "cabinet_W_door_LR_length = cabinet_W_side_length - ( cabinet_W_door_offset * 2 ) - ( cabinet_W_door_TB_width * 2 )"
equation "d244 = cabinet_W_door_TB_length"
equation "d245 = cabinet_W_door_TB_width"
equation "cabinet_door_bezzle = 2 in"
equation "d247 = material_thickness"
equation "d251 = -cabinet_W_front_LR_length - ( cabinet_W_door_TB_width * 2 ) + ( cabinet_W_door_offset * 2 )"
equation "d255 = -( cabinet_W_front_TB_length - cabinet_W_door_TB_length - ( cabinet_W_door_offset * 2 ) )"
equation "cabinet_W_door_LR_width = cabinet_door_bezzle"
equation "d258 = cabinet_W_door_LR_width"
equation "d259 = cabinet_W_door_LR_length"
equation "d260 = -material_thickness"
equation "d264 = -( cabinet_W_door_TB_length - cabinet_W_door_LR_width )"
equation "cabinet_W_door_rabbit = material_door_center"
equation "cabinet_W_door_center_width = cabinet_W_door_TB_length - ( cabinet_W_door_LR_width * 2 ) + ( cabinet_W_door_rabbit )"
equation "cabinet_W_door_center_length = cabinet_W_door_LR_length + cabinet_W_door_rabbit"
equation "d269 = cabinet_W_door_rabbit / 2"
equation "d270 = cabinet_W_door_rabbit / 2"
equation "d271 = cabinet_W_door_center_width"
equation "d272 = cabinet_W_door_center_length"
equation "cabinet_W_door_center_thickness = material_door_center"
equation "material_door_center = 0.25 in"
equation "d275 = -cabinet_W_door_center_thickness"
equation "d277 = shlf_W_NumOfSections"
equation "d279 = cabinet_W_front_TB_length"
equation "cabinet_W_trim_W_length = cabinet_W_tblTopLength + material_thickness" comment "material thickness is to accomidate for champher"
equation "cabinet_W_trim_W_width = material_thickness + cabinet_W_door_offset - 0.25 in"
equation "d283 = cabinet_W_trim_W_length"
equation "d284 = cabinet_W_trim_W_width"
equation "d285 = material_thickness"
equation "d287 = material_thickness"
equation "cabinet_W_trim_N_length = cabinet_depth + material_thickness"
equation "cabinet_W_trim_N_width = cabinet_W_trim_W_width" comment "b/c it needs to match the other trim"
equation "d290 = cabinet_W_trim_N_length"
equation "d291 = cabinet_W_trim_N_width"
equation "d292 = material_thickness"
equation "d294 = material_thickness"
equation "d297 = cabinet_height - ( cabinet_W_trim_N_width / 2 ) - 0.25 in"
equation "shlf_W_molding_width = 1.5 in"
equation "shlf_W_molding_length = shlf_W_side_length"
equation "shlf_W_molding_origin = 0.001 in"
equation "d302 = shlf_W_molding_origin"
equation "d303 = shlf_W_molding_width"
equation "d304 = shlf_W_molding_length"
equation "d305 = shlf_W_molding_width"
equation "d306 = shlf_W_molding_length"
equation "d307 = cabinet_W_tblTopLength"
equation "d308 = material_thickness"
equation "d314 = cabinet_W_tblTopLength - shlf_W_molding_width"
equation "d316 = cabinet_W_trim_W_width - material_thickness"
equation "cabinet_W_trim_W_LR_length = ( cabinet_W_front_width * 2 ) + cabinet_W_front_LR_length - ( cabinet_W_trim_W_LR_width * 2 )"
equation "cabinet_W_trim_W_LR_width = shlf_W_molding_width"
equation "d319 = cabinet_W_trim_W_LR_length"
equation "d320 = cabinet_W_trim_W_LR_width"
